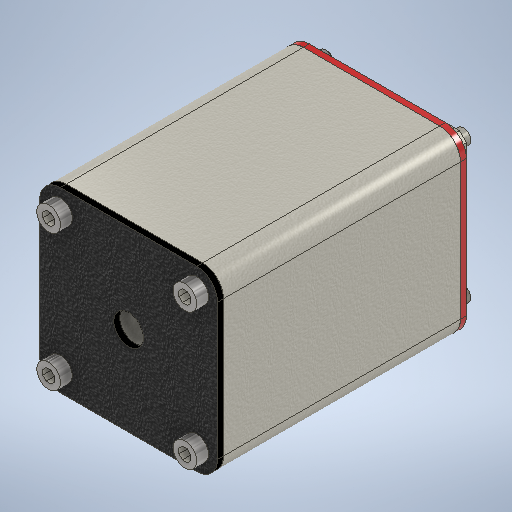
# Autodesk Inventor part: Part6
Saved by Autodesk Inventor 2025 (Build 290162000, 162)
## iProperties
Created: 2026-06-07
Part Number: Part6
Material: Generic
Document SubType Name: Modeling
Designer: user
Density: 1 g/cm^3
Appearance: Steel - Cast
Author: user
Autodesk Inventor part; units mm, degrees
ref_plane "YZ Plane" through (0, 0, 0) normal (1, 0, 0) x (0, 1, 0)
ref_plane "XZ Plane" through (0, 0, 0) normal (0, 1, 0) x (-1, 0, 0)
ref_plane "XY Plane" through (0, 0, 0) normal (0, 0, 1) x (1, 0, 0)
sketch "Sketch1" plane through (0, 0, 0) normal (0, 0, 1) x (1, 0, 0)
  line L0 (30, 30) -> (-30, 30)
  line L1 (-30, 30) -> (-30, -30)
  line L2 (-30, -30) -> (30, -30)
  line L3 (30, -30) -> (30, 30)
  line L4 (30, 30) -> (-30, -30) construction
  line L5 (-30, 30) -> (30, -30) construction
  point P0 (0, 0)
  dimension "d0" = 60
  dimension "d1" = 60
  constraints: 12 end point, 2 midpoint, 2 parallel, 1 horizontal, 1 perpendicular
  measures "d0" distance of L2.end L1.end
  measures "d1" distance of L2.end L0.start
extrude "Extrusion1" add sketch "Sketch1" along normal blind 80
fillet "Fillet1" radius 7 4 edges at (30, -30, 40) (30, 30, 40) (-30, -30, 40) (-30, 30, 40)
sketch "Sketch2" plane through (0, 0, 0) normal (0, 0, -1) x (-1, 0, 0)
  arc A0 (-23, 30) -> (-30, 23) centre (-23, 23) ccw projected
  circle A1 centre (-23, 23) radius 2.5
  arc A2 (30, 23) -> (23, 30) centre (23, 23) ccw projected
  circle A3 centre (23, 23) radius 2.5
  arc A4 (-30, -23) -> (-23, -30) centre (-23, -23) ccw projected
  circle A5 centre (-23, -23) radius 2.5
  arc A6 (23, -30) -> (30, -23) centre (23, -23) ccw projected
  circle A7 centre (23, -23) radius 2.5
  point P0 (0, 0)
  dimension "d5" = 5
  dimension "d6" = 5
  dimension "d7" = 5
  dimension "d8" = 5
  constraints: 4 centre point, 4 coincident
  measures "d5" diameter of A1
  measures "d6" diameter of A3
  measures "d7" diameter of A5
  measures "d8" diameter of A7
extrude "Extrusion2" cut sketch "Sketch2" against normal blind 80
sketch "Sketch3" plane through (0, 0, 80) normal (0, 0, 1) x (1, 0, 0)
  circle A0 centre (0, 0) radius 5
  dimension "d11" = 10
  constraints: 1 centre point, 1 coincident
  measures "d11" diameter of A0
extrude "Extrusion3" cut sketch "Sketch3" against normal blind 50
sketch "Sketch4" plane through (0, 0, 80) normal (0, 0, 1) x (1, 0, 0)
  circle A0 centre (0, 0) radius 5 projected
  circle A1 centre (23, -23) radius 2.5 projected
  circle A2 centre (-23, 23) radius 2.5 projected
  circle A3 centre (-23, -23) radius 2.5 projected
  circle A4 centre (23, 23) radius 2.5 projected
  arc A5 (-23, 30) -> (-30, 23) centre (-23, 23) ccw projected
  line L0 (-30, 23) -> (-30, -23) projected
  arc A6 (-30, -23) -> (-23, -30) centre (-23, -23) ccw projected
  line L1 (-23, -30) -> (23, -30) projected
  arc A7 (23, -30) -> (30, -23) centre (23, -23) ccw projected
  line L2 (30, -23) -> (30, 23) projected
  arc A8 (30, 23) -> (23, 30) centre (23, 23) ccw projected
  line L3 (23, 30) -> (-23, 30) projected
extrude "Extrusion4" add sketch "Sketch4" along normal blind 2 separate body
sketch "Sketch5" plane through (0, 0, 0) normal (0, 0, -1) x (-1, 0, 0)
  circle A0 centre (-23, -23) radius 2.5 projected
  circle A1 centre (23, 23) radius 2.5 projected
  circle A2 centre (23, -23) radius 2.5 projected
  circle A3 centre (-23, 23) radius 2.5 projected
  arc A4 (30, 23) -> (23, 30) centre (23, 23) ccw projected
  line L0 (-23, 30) -> (23, 30) projected
  arc A5 (-23, 30) -> (-30, 23) centre (-23, 23) ccw projected
  line L1 (-30, -23) -> (-30, 23) projected
  arc A6 (-30, -23) -> (-23, -30) centre (-23, -23) ccw projected
  line L2 (23, -30) -> (-23, -30) projected
  arc A7 (23, -30) -> (30, -23) centre (23, -23) ccw projected
  line L3 (30, 23) -> (30, -23) projected
  point P0 (0, 0)
extrude "Extrusion5" add sketch "Sketch5" along normal blind 2 separate body
sketch "Sketch6" plane through (0, 0, 82) normal (0, 0, 1) x (1, 0, 0)
  circle A0 centre (23, 23) radius 2.5 projected
  circle A1 centre (23, 23) radius 4
  point P0 (0, 0)
  dimension "d18" = 8
  constraints: 1 centre point, 1 coincident
  measures "d18" diameter of A1
extrude "Extrusion6" add sketch "Sketch6" along normal blind 4 separate body contours A0 | A1
sketch "Sketch7" plane through (23, 23, 86) normal (0, 0, 1) x (1, 0, 0)
  line L0 (2, 2) -> (-2, 2)
  line L1 (-2, 2) -> (-2, -2)
  line L2 (-2, -2) -> (2, -2)
  line L3 (2, -2) -> (2, 2)
  line L4 (2, 2) -> (-2, -2) construction
  line L5 (-2, 2) -> (2, -2) construction
  line L6 (-3.4142, 0.5858) -> (0.5858, -3.4142)
  line L7 (-0.5858, 3.4142) -> (3.4142, -0.5858)
  line L8 (0.5858, 3.4142) -> (-3.4142, -0.5858)
  line L9 (3.4142, 0.5858) -> (-0.5858, -3.4142)
  line L10 (2, 2) -> (1.4142, 1.4142)
  line L11 (-1.4142, -1.4142) -> (-2, -2)
  line L12 (2, -2) -> (1.4142, -1.4142)
  line L13 (-1.4142, 1.4142) -> (-2, 2)
  point P0 (-23, -23)
  point P1 (2, -0.8284)
  point P2 (2, 0.8284)
  point P3 (0.8284, 2)
  point P4 (-0.8284, 2)
  point P5 (-2, 0.8284)
  point P6 (-2, -0.8284)
  point P7 (-0.8284, -2)
  point P8 (0.8284, -2)
  dimension "d21" = 4
  dimension "d22" = 4
  dimension "d23" = 2
  dimension "d24" = 4
  dimension "d25" = 2
  dimension "d26" = 4
  constraints: 28 end point, 6 parallel, 4 midpoint, 2 collinear, 1 horizontal, 1 perpendicular
  measures "d21" distance of L2.end L1.end
  measures "d22" distance of L1.end L0.end
  measures "d23" distance between parallel lines of L5 L6
  measures "d24" distance between parallel lines of L6 L7
  measures "d25" distance between parallel lines of L4 L8
  measures "d26" distance between parallel lines of L8 L9
extrude "Extrusion7" cut sketch "Sketch7" against normal blind 3 contours L7 L3 L9 L2 L6 L1 L8 L0 bodies 4
pattern_circular "Circular Pattern1" count 4 over 360 about axis through (0, 0, 80) along (0, 0, 1) of "Extrusion6" bodies 4
pattern_circular "Circular Pattern2" count 4 over 360 about axis through (0, 0, 80) along (0, 0, 1) of "Extrusion7" bodies 4
sketch "Sketch8" plane through (0, 0, -2) normal (0, 0, -1) x (-1, 0, 0)
  line L0 (27, 27) -> (19, 27)
  line L1 (19, 27) -> (19, 19)
  line L2 (19, 19) -> (27, 19)
  line L3 (27, 19) -> (27, 27)
  circle A0 centre (23, 23) radius 2.5 projected
  line L4 (27, 27) -> (19, 19) construction
  line L5 (19, 27) -> (27, 19) construction
  line L6 (24.1716, 29.8284) -> (16.1716, 21.8284)
  line L7 (29.8284, 24.1716) -> (21.8284, 16.1716)
  line L8 (16.1716, 24.1716) -> (24.1716, 16.1716)
  line L9 (21.8284, 29.8284) -> (29.8284, 21.8284)
  line L10 (27, 27) -> (25.8284, 25.8284)
  line L11 (21.2322, 24.7678) -> (19, 27)
  line L12 (24.7678, 24.7678) -> (23, 23)
  line L13 (21.2322, 21.2322) -> (19, 19)
  line L14 (27, 19) -> (25.8284, 20.1716)
  line L15 (24.7678, 21.2322) -> (23, 23)
  point P0 (0, 0)
  point P1 (19, 24.6569)
  point P2 (19, 21.3431)
  point P3 (21.3431, 19)
  point P4 (24.6569, 19)
  point P5 (27, 21.3431)
  point P6 (27, 24.6569)
  point P7 (24.6569, 27)
  point P8 (21.3431, 27)
  dimension "d35" = 4
  dimension "d36" = 8
  dimension "d37" = 4
  dimension "d38" = 8
  constraints: 32 end point, 10 perpendicular, 6 midpoint, 6 parallel, 4 point on circle, 3 collinear, 1 horizontal
  measures "d35" distance between parallel lines of L4 L6
  measures "d36" distance between parallel lines of L6 L7
  measures "d37" distance between parallel lines of L5 L8
  measures "d38" distance between parallel lines of L8 L9
extrude "Extrusion8" add sketch "Sketch8" along normal blind 3 separate body contours L9 L3 L7 L2 L8 L13 A0 L11 L6 L0 | L11 A0 L13 L8 L1 L6
sketch "Sketch9" plane through (0, 0, -5) normal (0, 0, -1) x (-1, 0, 0)
  circle A0 centre (23, 23) radius 2.5 projected
  point P0 (0, 0)
extrude "Extrusion9" add sketch "Sketch9" along normal blind 3 bodies 5
chamfer "Chamfer1" distance 0.5 angle 45 1 edges at (-20.5, 23, -8)
thread "Thread1" size "M5x0.8" class "6g" standard "ANSI Metric M Profile" length 60
pattern_circular "Circular Pattern3" count 4 over 360 about axis through (0, 0, 80) along (0, 0, 1) of "Extrusion8", "Extrusion9" bodies 5
body "Solid1"
body "Solid2"
body "Solid3"
body "Solid4"
body "Solid6"
body "Solid7"
